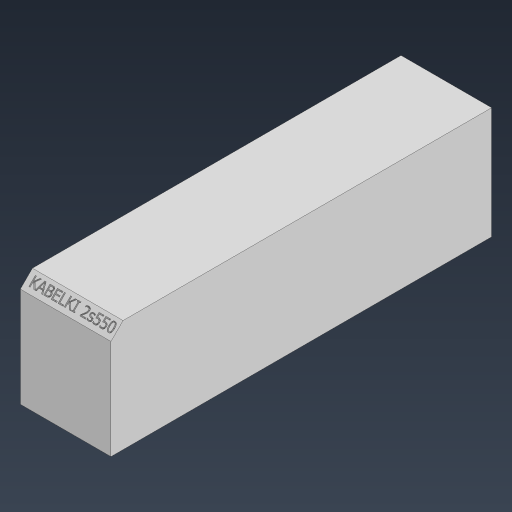
# Autodesk Inventor part: 2s450mah
Saved by Autodesk Inventor 2023 (Build 270158000, 158)
## iProperties
Created: 2026-03-09
Part Number: 2s450mah
Material: Generic
Document SubType Name: Modeling
Designer: szymo
Density: 1 g/cm^3
Appearance: Default
Author: szymo
Autodesk Inventor part; units mm, degrees
ref_plane "YZ Plane" through (0, 0, 0) normal (1, 0, 0) x (0, 1, 0)
ref_plane "XZ Plane" through (0, 0, 0) normal (0, 1, 0) x (-1, 0, 0)
ref_plane "XY Plane" through (0, 0, 0) normal (0, 0, 1) x (1, 0, 0)
sketch "Sketch1" plane through (0, 0, 0) normal (0, 1, 0) x (-1, 0, 0)
  line L0 (0, 0) -> (-15, 0)
  line L1 (-15, 0) -> (-15, -63)
  line L2 (-15, -63) -> (0, -63)
  line L3 (0, -63) -> (0, 0)
  dimension "d0" = 15
  dimension "d1" = 63
  constraints: 8 end point, 2 parallel, 1 horizontal, 1 perpendicular
  measures "d0" distance of L2.end L1.end
  measures "d1" distance of L0.end L1.end
extrude "Extrusion1" add sketch "Sketch1" along normal blind 18.5
chamfer "Chamfer1" distance 2 angle 45 1 edges at (7.5, 18.5, 0)
sketch "Sketch2" plane through (0, 18.5, -2) normal (0, 0.7071068, 0.7071068) x (1, 0, 0)
  line L0 (0.7167, -0.5374) -> (24.0854, -0.5374) construction
  line L1 (24.0854, -0.5374) -> (24.0854, -3.5854) construction
  line L2 (24.0854, -3.5854) -> (0.7167, -3.5854) construction
  line L3 (0.7167, -3.5854) -> (0.7167, -0.5374) construction
  line L4 (1.9626, -2.069) -> (1.7037, -2.069)
  line L5 (1.7037, -2.069) -> (1.1555, -1.3713)
  line L6 (1.1555, -1.3713) -> (1.068, -1.4698)
  line L7 (1.068, -1.4698) -> (1.068, -2.069)
  line L8 (1.068, -2.069) -> (0.8686, -2.069)
  line L9 (0.8686, -2.069) -> (0.8686, -0.569)
  line L10 (0.8686, -0.569) -> (1.068, -0.569)
  line L11 (1.068, -0.569) -> (1.068, -1.2583)
  line L12 (1.068, -1.2583) -> (1.683, -0.569)
  line L13 (1.683, -0.569) -> (1.9262, -0.569)
  line L14 (1.9262, -0.569) -> (1.305, -1.2388)
  line L15 (1.305, -1.2388) -> (1.9626, -2.069)
  line L16 (1.9201, -2.069) -> (2.4257, -0.569)
  line L17 (2.4257, -0.569) -> (2.6713, -0.569)
  line L18 (2.6713, -0.569) -> (3.177, -2.069)
  line L19 (3.177, -2.069) -> (2.9667, -2.069)
  line L20 (2.9667, -2.069) -> (2.8305, -1.6497)
  line L21 (2.8305, -1.6497) -> (2.258, -1.6497)
  line L22 (2.258, -1.6497) -> (2.1219, -2.069)
  line L23 (2.1219, -2.069) -> (1.9201, -2.069)
  line L24 (2.7758, -1.4795) -> (2.5437, -0.7733)
  line L25 (2.5437, -0.7733) -> (2.3127, -1.4795)
  line L26 (2.3127, -1.4795) -> (2.7758, -1.4795)
  spline S0 degree 2 poles (4.3366, -1.6083) (4.3366, -1.7202) (4.2515, -1.8916) (4.181, -1.9475) knots 0 0 0 1 2 2 2
  spline S1 degree 2 poles (4.181, -1.9475) (4.0959, -2.0131) (3.9027, -2.069) (3.7495, -2.069) knots 0 0 0 1 2 2 2
  line L27 (3.7495, -2.069) -> (3.3192, -2.069)
  line L28 (3.3192, -2.069) -> (3.3192, -0.569)
  line L29 (3.3192, -0.569) -> (3.7167, -0.569)
  spline S2 degree 2 poles (3.7167, -0.569) (3.8771, -0.569) (4.0376, -0.5897) (4.1105, -0.6298) knots 0 0 0 1 2 2 2
  spline S3 degree 2 poles (4.1105, -0.6298) (4.192, -0.6724) (4.2661, -0.8121) (4.2661, -0.907) knots 0 0 0 1 2 2 2
  spline S4 degree 2 poles (4.2661, -0.907) (4.2661, -1.0127) (4.1543, -1.1805) (4.0558, -1.2279) knots 0 0 0 1 2 2 2
  line L30 (4.0558, -1.2279) -> (4.0558, -1.2352)
  spline S5 degree 2 poles (4.0558, -1.2352) (4.1895, -1.2716) (4.3366, -1.4649) (4.3366, -1.6083) knots 0 0 0 1 2 2 2
  spline S6 degree 2 poles (4.1287, -1.6168) (4.1287, -1.5318) (4.0801, -1.4224) (4.0072, -1.3835) knots 0 0 0 1 2 2 2
  spline S7 degree 2 poles (4.0072, -1.3835) (3.9598, -1.3591) (3.848, -1.3446) (3.7446, -1.3446) knots 0 0 0 1 2 2 2
  line L31 (3.7446, -1.3446) -> (3.5185, -1.3446)
  line L32 (3.5185, -1.3446) -> (3.5185, -1.8989)
  line L33 (3.5185, -1.8989) -> (3.6802, -1.8989)
  spline S8 degree 2 poles (3.6802, -1.8989) (3.8115, -1.8989) (3.9622, -1.8745) (4.0206, -1.8356) knots 0 0 0 1 2 2 2
  spline S9 degree 2 poles (4.0206, -1.8356) (4.0765, -1.7955) (4.1287, -1.6959) (4.1287, -1.6168) knots 0 0 0 1 2 2 2
  spline S10 degree 2 poles (4.0582, -0.9349) (4.0582, -0.8814) (4.0218, -0.8012) (3.9817, -0.7781) knots 0 0 0 1 2 2 2
  spline S11 degree 2 poles (3.9817, -0.7781) (3.933, -0.7514) (3.8151, -0.7392) (3.7094, -0.7392) knots 0 0 0 1 2 2 2
  line L34 (3.7094, -0.7392) -> (3.5185, -0.7392)
  line L35 (3.5185, -0.7392) -> (3.5185, -1.178)
  line L36 (3.5185, -1.178) -> (3.7446, -1.178)
  spline S12 degree 2 poles (3.7446, -1.178) (3.8382, -1.178) (3.927, -1.1586) (3.9744, -1.1282) knots 0 0 0 1 2 2 2
  spline S13 degree 2 poles (3.9744, -1.1282) (4.0206, -1.099) (4.0582, -1.0054) (4.0582, -0.9349) knots 0 0 0 1 2 2 2
  line L37 (4.5347, -2.069) -> (4.5347, -0.569)
  line L38 (4.5347, -0.569) -> (5.4732, -0.569)
  line L39 (5.4732, -0.569) -> (5.4732, -0.7465)
  line L40 (5.4732, -0.7465) -> (4.7341, -0.7465)
  line L41 (4.7341, -0.7465) -> (4.7341, -1.1574)
  line L42 (4.7341, -1.1574) -> (5.4233, -1.1574)
  line L43 (5.4233, -1.1574) -> (5.4233, -1.3348)
  line L44 (5.4233, -1.3348) -> (4.7341, -1.3348)
  line L45 (4.7341, -1.3348) -> (4.7341, -1.8916)
  line L46 (4.7341, -1.8916) -> (5.4732, -1.8916)
  line L47 (5.4732, -1.8916) -> (5.4732, -2.069)
  line L48 (5.4732, -2.069) -> (4.5347, -2.069)
  line L49 (6.5611, -2.069) -> (5.692, -2.069)
  line L50 (5.692, -2.069) -> (5.692, -0.569)
  line L51 (5.692, -0.569) -> (5.8913, -0.569)
  line L52 (5.8913, -0.569) -> (5.8913, -1.8916)
  line L53 (5.8913, -1.8916) -> (6.5611, -1.8916)
  line L54 (6.5611, -1.8916) -> (6.5611, -2.069)
  line L55 (7.8119, -2.069) -> (7.553, -2.069)
  line L56 (7.553, -2.069) -> (7.0048, -1.3713)
  line L57 (7.0048, -1.3713) -> (6.9172, -1.4698)
  line L58 (6.9172, -1.4698) -> (6.9172, -2.069)
  line L59 (6.9172, -2.069) -> (6.7179, -2.069)
  line L60 (6.7179, -2.069) -> (6.7179, -0.569)
  line L61 (6.7179, -0.569) -> (6.9172, -0.569)
  line L62 (6.9172, -0.569) -> (6.9172, -1.2583)
  line L63 (6.9172, -1.2583) -> (7.5323, -0.569)
  line L64 (7.5323, -0.569) -> (7.7754, -0.569)
  line L65 (7.7754, -0.569) -> (7.1543, -1.2388)
  line L66 (7.1543, -1.2388) -> (7.8119, -2.069)
  line L67 (8.4537, -2.069) -> (7.8727, -2.069)
  line L68 (7.8727, -2.069) -> (7.8727, -1.9159)
  line L69 (7.8727, -1.9159) -> (8.0635, -1.9159)
  line L70 (8.0635, -1.9159) -> (8.0635, -0.7222)
  line L71 (8.0635, -0.7222) -> (7.8727, -0.7222)
  line L72 (7.8727, -0.7222) -> (7.8727, -0.569)
  line L73 (7.8727, -0.569) -> (8.4537, -0.569)
  line L74 (8.4537, -0.569) -> (8.4537, -0.7222)
  line L75 (8.4537, -0.7222) -> (8.2629, -0.7222)
  line L76 (8.2629, -0.7222) -> (8.2629, -1.9159)
  line L77 (8.2629, -1.9159) -> (8.4537, -1.9159)
  line L78 (8.4537, -1.9159) -> (8.4537, -2.069)
  line L79 (10.2272, -2.069) -> (9.3022, -2.069)
  line L80 (9.3022, -2.069) -> (9.3022, -1.8563)
  spline S14 degree 2 poles (9.3022, -1.8563) (9.4018, -1.7627) (9.5793, -1.5889) (9.6644, -1.4953) knots 0 0 0 1 2 2 2
  spline S15 degree 2 poles (9.6644, -1.4953) (9.8358, -1.3069) (9.961, -1.0808) (9.961, -0.9604) knots 0 0 0 1 2 2 2
  spline S16 degree 2 poles (9.961, -0.9604) (9.961, -0.8972) (9.9221, -0.8024) (9.8868, -0.772) knots 0 0 0 1 2 2 2
  spline S17 degree 2 poles (9.8868, -0.772) (9.8516, -0.7416) (9.7592, -0.7113) (9.7033, -0.7113) knots 0 0 0 1 2 2 2
  spline S18 degree 2 poles (9.7033, -0.7113) (9.6498, -0.7113) (9.5404, -0.738) (9.4906, -0.7587) knots 0 0 0 1 2 2 2
  spline S19 degree 2 poles (9.4906, -0.7587) (9.448, -0.7757) (9.369, -0.8243) (9.3447, -0.8413) knots 0 0 0 1 2 2 2
  line L81 (9.3447, -0.8413) -> (9.3338, -0.8413)
  line L82 (9.3338, -0.8413) -> (9.3338, -0.6274)
  spline S20 degree 2 poles (9.3338, -0.6274) (9.3958, -0.597) (9.6182, -0.5374) (9.7179, -0.5374) knots 0 0 0 1 2 2 2
  spline S21 degree 2 poles (9.7179, -0.5374) (9.9282, -0.5374) (10.1652, -0.7599) (10.1652, -0.9495) knots 0 0 0 1 2 2 2
  spline S22 degree 2 poles (10.1652, -0.9495) (10.1652, -1.0382) (10.1239, -1.1865) (10.0874, -1.2497) knots 0 0 0 1 2 2 2
  spline S23 degree 2 poles (10.0874, -1.2497) (10.0509, -1.3154) (9.9452, -1.4442) (9.8868, -1.5062) knots 0 0 0 1 2 2 2
  spline S24 degree 2 poles (9.8868, -1.5062) (9.792, -1.6096) (9.5599, -1.8308) (9.4906, -1.8952) knots 0 0 0 1 2 2 2
  line L83 (9.4906, -1.8952) -> (10.2272, -1.8952)
  line L84 (10.2272, -1.8952) -> (10.2272, -2.069)
  spline S25 degree 2 poles (10.7596, -2.0958) (10.6466, -2.0958) (10.4509, -2.035) (10.3864, -2.001) knots 0 0 0 1 2 2 2
  line L85 (10.3864, -2.001) -> (10.3864, -1.7882)
  line L86 (10.3864, -1.7882) -> (10.3962, -1.7882)
  spline S26 degree 2 poles (10.3962, -1.7882) (10.4205, -1.8077) (10.4861, -1.8539) (10.5408, -1.8794) knots 0 0 0 1 2 2 2
  spline S27 degree 2 poles (10.5408, -1.8794) (10.5882, -1.9025) (10.7049, -1.9365) (10.7669, -1.9365) knots 0 0 0 1 2 2 2
  spline S28 degree 2 poles (10.7669, -1.9365) (10.8119, -1.9365) (10.9152, -1.9159) (10.9395, -1.8989) knots 0 0 0 1 2 2 2
  spline S29 degree 2 poles (10.9395, -1.8989) (10.9748, -1.8758) (11.0064, -1.8235) (11.0064, -1.77) knots 0 0 0 1 2 2 2
  spline S30 degree 2 poles (11.0064, -1.77) (11.0064, -1.7032) (10.9334, -1.6339) (10.8398, -1.6108) knots 0 0 0 1 2 2 2
  spline S31 degree 2 poles (10.8398, -1.6108) (10.8034, -1.6023) (10.6867, -1.578) (10.6368, -1.5646) knots 0 0 0 1 2 2 2
  spline S32 degree 2 poles (10.6368, -1.5646) (10.508, -1.5269) (10.3913, -1.3713) (10.3913, -1.2607) knots 0 0 0 1 2 2 2
  spline S33 degree 2 poles (10.3913, -1.2607) (10.3913, -1.1075) (10.621, -0.9167) (10.8107, -0.9167) knots 0 0 0 1 2 2 2
  spline S34 degree 2 poles (10.8107, -0.9167) (10.9043, -0.9167) (11.0939, -0.9629) (11.1583, -0.9981) knots 0 0 0 1 2 2 2
  line L87 (11.1583, -0.9981) -> (11.1583, -1.2011)
  line L88 (11.1583, -1.2011) -> (11.1486, -1.2011)
  spline S35 degree 2 poles (11.1486, -1.2011) (11.0757, -1.1428) (10.8982, -1.0759) (10.807, -1.0759) knots 0 0 0 1 2 2 2
  spline S36 degree 2 poles (10.807, -1.0759) (10.7134, -1.0759) (10.5846, -1.1549) (10.5846, -1.2339) knots 0 0 0 1 2 2 2
  spline S37 degree 2 poles (10.5846, -1.2339) (10.5846, -1.3057) (10.6612, -1.375) (10.7462, -1.3968) knots 0 0 0 1 2 2 2
  spline S38 degree 2 poles (10.7462, -1.3968) (10.7876, -1.4078) (10.8921, -1.4297) (10.9492, -1.443) knots 0 0 0 1 2 2 2
  spline S39 degree 2 poles (10.9492, -1.443) (11.0732, -1.4746) (11.1997, -1.6193) (11.1997, -1.7445) knots 0 0 0 1 2 2 2
  spline S40 degree 2 poles (11.1997, -1.7445) (11.1997, -1.8174) (11.1425, -1.9463) (11.0866, -1.9937) knots 0 0 0 1 2 2 2
  spline S41 degree 2 poles (11.0866, -1.9937) (11.027, -2.0435) (10.8751, -2.0958) (10.7596, -2.0958) knots 0 0 0 1 2 2 2
  spline S42 degree 2 poles (12.2572, -1.5925) (12.2572, -1.7007) (12.1879, -1.8855) (12.1247, -1.9536) knots 0 0 0 1 2 2 2
  spline S43 degree 2 poles (12.1247, -1.9536) (12.0615, -2.0216) (11.8731, -2.1006) (11.7564, -2.1006) knots 0 0 0 1 2 2 2
  spline S44 degree 2 poles (11.7564, -2.1006) (11.6494, -2.1006) (11.4403, -2.0532) (11.3638, -2.0156) knots 0 0 0 1 2 2 2
  line L89 (11.3638, -2.0156) -> (11.3638, -1.8028)
  line L90 (11.3638, -1.8028) -> (11.3783, -1.8028)
  spline S45 degree 2 poles (11.3783, -1.8028) (11.4014, -1.8198) (11.4877, -1.8636) (11.54, -1.8831) knots 0 0 0 1 2 2 2
  spline S46 degree 2 poles (11.54, -1.8831) (11.5996, -1.9037) (11.698, -1.9268) (11.76, -1.9268) knots 0 0 0 1 2 2 2
  spline S47 degree 2 poles (11.76, -1.9268) (11.8208, -1.9268) (11.9351, -1.8831) (11.9764, -1.8356) knots 0 0 0 1 2 2 2
  spline S48 degree 2 poles (11.9764, -1.8356) (12.0141, -1.7907) (12.053, -1.6715) (12.053, -1.5913) knots 0 0 0 1 2 2 2
  spline S49 degree 2 poles (12.053, -1.5913) (12.053, -1.5111) (12.0092, -1.409) (11.9679, -1.375) knots 0 0 0 1 2 2 2
  spline S50 degree 2 poles (11.9679, -1.375) (11.9253, -1.3373) (11.7989, -1.3057) (11.7223, -1.3057) knots 0 0 0 1 2 2 2
  spline S51 degree 2 poles (11.7223, -1.3057) (11.6397, -1.3057) (11.4756, -1.3312) (11.4257, -1.3421) knots 0 0 0 1 2 2 2
  line L91 (11.4257, -1.3421) -> (11.4257, -0.569)
  line L92 (11.4257, -0.569) -> (12.2487, -0.569)
  line L93 (12.2487, -0.569) -> (12.2487, -0.7453)
  line L94 (12.2487, -0.7453) -> (11.619, -0.7453)
  line L95 (11.619, -0.7453) -> (11.619, -1.1452)
  spline S52 degree 2 poles (11.619, -1.1452) (11.6555, -1.1403) (11.726, -1.1367) (11.7552, -1.1367) knots 0 0 0 1 2 2 2
  spline S53 degree 2 poles (11.7552, -1.1367) (11.8706, -1.1367) (12.0299, -1.1744) (12.1028, -1.2303) knots 0 0 0 1 2 2 2
  spline S54 degree 2 poles (12.1028, -1.2303) (12.177, -1.2862) (12.2572, -1.4564) (12.2572, -1.5925) knots 0 0 0 1 2 2 2
  spline S55 degree 2 poles (13.3828, -1.5925) (13.3828, -1.7007) (13.3135, -1.8855) (13.2503, -1.9536) knots 0 0 0 1 2 2 2
  spline S56 degree 2 poles (13.2503, -1.9536) (13.1871, -2.0216) (12.9987, -2.1006) (12.882, -2.1006) knots 0 0 0 1 2 2 2
  spline S57 degree 2 poles (12.882, -2.1006) (12.775, -2.1006) (12.5659, -2.0532) (12.4894, -2.0156) knots 0 0 0 1 2 2 2
  line L96 (12.4894, -2.0156) -> (12.4894, -1.8028)
  line L97 (12.4894, -1.8028) -> (12.5039, -1.8028)
  spline S58 degree 2 poles (12.5039, -1.8028) (12.527, -1.8198) (12.6133, -1.8636) (12.6656, -1.8831) knots 0 0 0 1 2 2 2
  spline S59 degree 2 poles (12.6656, -1.8831) (12.7252, -1.9037) (12.8236, -1.9268) (12.8856, -1.9268) knots 0 0 0 1 2 2 2
  spline S60 degree 2 poles (12.8856, -1.9268) (12.9464, -1.9268) (13.0607, -1.8831) (13.102, -1.8356) knots 0 0 0 1 2 2 2
  spline S61 degree 2 poles (13.102, -1.8356) (13.1397, -1.7907) (13.1786, -1.6715) (13.1786, -1.5913) knots 0 0 0 1 2 2 2
  spline S62 degree 2 poles (13.1786, -1.5913) (13.1786, -1.5111) (13.1348, -1.409) (13.0935, -1.375) knots 0 0 0 1 2 2 2
  spline S63 degree 2 poles (13.0935, -1.375) (13.0509, -1.3373) (12.9245, -1.3057) (12.848, -1.3057) knots 0 0 0 1 2 2 2
  spline S64 degree 2 poles (12.848, -1.3057) (12.7653, -1.3057) (12.6012, -1.3312) (12.5514, -1.3421) knots 0 0 0 1 2 2 2
  line L98 (12.5514, -1.3421) -> (12.5514, -0.569)
  line L99 (12.5514, -0.569) -> (13.3743, -0.569)
  line L100 (13.3743, -0.569) -> (13.3743, -0.7453)
  line L101 (13.3743, -0.7453) -> (12.7446, -0.7453)
  line L102 (12.7446, -0.7453) -> (12.7446, -1.1452)
  spline S65 degree 2 poles (12.7446, -1.1452) (12.7811, -1.1403) (12.8516, -1.1367) (12.8808, -1.1367) knots 0 0 0 1 2 2 2
  spline S66 degree 2 poles (12.8808, -1.1367) (12.9962, -1.1367) (13.1555, -1.1744) (13.2284, -1.2303) knots 0 0 0 1 2 2 2
  spline S67 degree 2 poles (13.2284, -1.2303) (13.3026, -1.2862) (13.3828, -1.4564) (13.3828, -1.5925) knots 0 0 0 1 2 2 2
  spline S68 degree 2 poles (14.5327, -1.319) (14.5327, -1.7226) (14.2981, -2.1006) (14.0538, -2.1006) knots 0 0 0 1 2 2 2
  spline S69 degree 2 poles (14.0538, -2.1006) (13.8058, -2.1006) (13.5736, -1.7153) (13.5736, -1.3203) knots 0 0 0 1 2 2 2
  spline S70 degree 2 poles (13.5736, -1.3203) (13.5736, -0.9143) (13.8082, -0.5386) (14.0538, -0.5386) knots 0 0 0 1 2 2 2
  spline S71 degree 2 poles (14.0538, -0.5386) (14.3005, -0.5386) (14.5327, -0.9276) (14.5327, -1.319) knots 0 0 0 1 2 2 2
  spline S72 degree 2 poles (14.275, -1.7761) (14.3042, -1.7019) (14.3285, -1.4734) (14.3285, -1.319) knots 0 0 0 1 2 2 2
  spline S73 degree 2 poles (14.3285, -1.319) (14.3285, -1.1647) (14.3042, -0.9374) (14.2738, -0.8608) knots 0 0 0 1 2 2 2
  spline S74 degree 2 poles (14.2738, -0.8608) (14.2434, -0.7842) (14.1377, -0.7052) (14.0538, -0.7052) knots 0 0 0 1 2 2 2
  spline S75 degree 2 poles (14.0538, -0.7052) (13.9699, -0.7052) (13.8617, -0.7842) (13.8301, -0.8632) knots 0 0 0 1 2 2 2
  spline S76 degree 2 poles (13.8301, -0.8632) (13.7997, -0.9398) (13.7779, -1.1732) (13.7779, -1.3203) knots 0 0 0 1 2 2 2
  spline S77 degree 2 poles (13.7779, -1.3203) (13.7779, -1.4783) (13.7973, -1.6898) (13.8289, -1.7724) knots 0 0 0 1 2 2 2
  spline S78 degree 2 poles (13.8289, -1.7724) (13.8581, -1.8502) (13.9663, -1.9341) (14.0538, -1.9341) knots 0 0 0 1 2 2 2
  spline S79 degree 2 poles (14.0538, -1.9341) (14.1364, -1.9341) (14.2446, -1.8551) (14.275, -1.7761) knots 0 0 0 1 2 2 2
  point P0 (0, -14.4957)
  constraints: 2 other
extrude "Extrusion2" cut sketch "Sketch2" against normal blind 1
body "Solid1"
